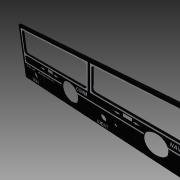
# Autodesk Inventor part: NavCom_panel
Saved by Autodesk Inventor 2014 (Build 180170000, 170)
## iProperties
Created: 2017-02-12
Part Number: NavCom_panel
Material: Všeobecné
Document SubType Name: Modeling
Designer: N
Density: 1 g/cm^3
Appearance: Výchozí
Author: N
Autodesk Inventor part; units mm, degrees
ref_plane "YZ Plane" through (0, 0, 0) normal (1, 0, 0) x (0, 1, 0)
ref_plane "XZ Plane" through (0, 0, 0) normal (0, 1, 0) x (-1, 0, 0)
ref_plane "XY Plane" through (0, 0, 0) normal (0, 0, 1) x (1, 0, 0)
sketch "Náčrt1" plane through (0, 0, 0) normal (0, 0, 1) x (1, 0, 0)
  circle A0 centre (29.21, 8.89) radius 2.54
  circle A1 centre (16.51, 8.89) radius 3.81
  circle A2 centre (65.405, 13.97) radius 10.795
  circle A3 centre (116.84, 8.89) radius 2.54
  circle A4 centre (104.14, 8.89) radius 3.81
  circle A5 centre (153.035, 13.97) radius 10.795
  line L0 (34.29, 25.7175) -> (44.45, 25.7175)
  line L1 (44.45, 25.7175) -> (44.45, 20.0025)
  line L2 (44.45, 20.0025) -> (34.29, 20.0025)
  line L3 (34.29, 20.0025) -> (34.29, 25.7175)
  line L4 (121.92, 25.7175) -> (132.08, 25.7175)
  line L5 (132.08, 25.7175) -> (132.08, 20.0025)
  line L6 (132.08, 20.0025) -> (121.92, 20.0025)
  line L7 (121.92, 20.0025) -> (121.92, 25.7175)
  line L8 (0, 55.88) -> (177.8, 55.88)
  line L9 (177.8, 55.88) -> (177.8, 0)
  line L10 (177.8, 0) -> (0, 0)
  line L11 (0, 0) -> (0, 55.88)
  line L12 (93.98, 52.07) -> (171.45, 52.07)
  arc A6 (173.99, 49.53) -> (171.45, 52.07) centre (171.45, 49.53) ccw
  line L13 (173.99, 49.53) -> (173.99, 30.48)
  arc A7 (171.45, 27.94) -> (173.99, 30.48) centre (171.45, 30.48) ccw
  line L14 (171.45, 27.94) -> (93.98, 27.94)
  arc A8 (91.44, 30.48) -> (93.98, 27.94) centre (93.98, 30.48) ccw
  line L15 (91.44, 30.48) -> (91.44, 49.53)
  arc A9 (93.98, 52.07) -> (91.44, 49.53) centre (93.98, 49.53) ccw
  line L16 (6.35, 52.07) -> (83.82, 52.07)
  arc A10 (86.36, 49.53) -> (83.82, 52.07) centre (83.82, 49.53) ccw
  line L17 (86.36, 49.53) -> (86.36, 30.48)
  arc A11 (83.82, 27.94) -> (86.36, 30.48) centre (83.82, 30.48) ccw
  line L18 (83.82, 27.94) -> (6.35, 27.94)
  arc A12 (3.81, 30.48) -> (6.35, 27.94) centre (6.35, 30.48) ccw
  line L19 (3.81, 30.48) -> (3.81, 49.53)
  arc A13 (6.35, 52.07) -> (3.81, 49.53) centre (6.35, 49.53) ccw
  constraints: 40 end point, 16 point on circle, 14 centre point
extrude "Vysunutí1" add sketch "Náčrt1" along normal blind 2.54
sketch "Náčrt2" plane through (0, 0, 2.54) normal (0, 0, 1) x (1, 0, 0)
  arc A0 (86.36, 49.53) -> (83.82, 52.07) centre (83.82, 49.53) ccw projected
  line L0 (86.36, 49.53) -> (86.36, 30.48) projected
  arc A1 (83.82, 27.94) -> (86.36, 30.48) centre (83.82, 30.48) ccw projected
  line L1 (83.82, 27.94) -> (6.35, 27.94) projected
  arc A2 (3.81, 30.48) -> (6.35, 27.94) centre (6.35, 30.48) ccw projected
  line L2 (3.81, 30.48) -> (3.81, 49.53) projected
  arc A3 (6.35, 52.07) -> (3.81, 49.53) centre (6.35, 49.53) ccw projected
  line L3 (6.35, 52.07) -> (83.82, 52.07) projected
  arc A4 (173.99, 49.53) -> (171.45, 52.07) centre (171.45, 49.53) ccw projected
  line L4 (173.99, 49.53) -> (173.99, 30.48) projected
  arc A5 (171.45, 27.94) -> (173.99, 30.48) centre (171.45, 30.48) ccw projected
  line L5 (171.45, 27.94) -> (93.98, 27.94) projected
  arc A6 (91.44, 30.48) -> (93.98, 27.94) centre (93.98, 30.48) ccw projected
  line L6 (91.44, 30.48) -> (91.44, 49.53) projected
  arc A7 (93.98, 52.07) -> (91.44, 49.53) centre (93.98, 49.53) ccw projected
  line L7 (93.98, 52.07) -> (171.45, 52.07) projected
  line L8 (0, 55.88) -> (177.8, 55.88)
  line L9 (177.8, 55.88) -> (177.8, 0)
  line L10 (177.8, 0) -> (0, 0)
  line L11 (0, 0) -> (0, 55.88)
  line L12 (74.93, 19.05) -> (143.51, 19.05)
  line L13 (162.56, 19.05) -> (171.45, 19.05)
  arc A8 (171.45, 19.05) -> (173.99, 21.59) centre (171.45, 21.59) ccw
  arc A9 (3.81, 21.59) -> (6.35, 19.05) centre (6.35, 21.59) ccw
  line L14 (87.63, 53.34) -> (2.54, 53.34)
  line L15 (6.35, 26.67) -> (87.63, 26.67)
  line L16 (2.54, 17.78) -> (2.54, 53.34)
  line L17 (3.81, 24.13) -> (3.81, 21.59)
  arc A10 (6.35, 26.67) -> (3.81, 24.13) centre (6.35, 24.13) ccw
  line L18 (90.17, 26.67) -> (171.45, 26.67)
  line L19 (175.26, 53.34) -> (90.17, 53.34)
  line L20 (90.17, 26.67) -> (90.17, 53.34)
  line L21 (87.63, 26.67) -> (87.63, 53.34)
  line L22 (175.26, 17.78) -> (175.26, 53.34)
  line L23 (173.99, 24.13) -> (173.99, 21.59)
  arc A11 (173.99, 24.13) -> (171.45, 26.67) centre (171.45, 24.13) ccw
  line L24 (175.26, 17.78) -> (163.1353, 17.78)
  line L25 (142.9347, 17.78) -> (75.5053, 17.78)
  line L26 (55.3047, 17.78) -> (2.54, 17.78)
  line L27 (6.35, 19.05) -> (55.88, 19.05)
  line L28 (93.98, 52.07) -> (171.45, 52.07)
  arc A12 (173.99, 49.53) -> (171.45, 52.07) centre (171.45, 49.53) ccw
  line L29 (173.99, 49.53) -> (173.99, 30.48)
  arc A13 (171.45, 27.94) -> (173.99, 30.48) centre (171.45, 30.48) ccw
  line L30 (171.45, 27.94) -> (93.98, 27.94)
  arc A14 (91.44, 30.48) -> (93.98, 27.94) centre (93.98, 30.48) ccw
  line L31 (91.44, 30.48) -> (91.44, 49.53)
  arc A15 (93.98, 52.07) -> (91.44, 49.53) centre (93.98, 49.53) ccw
  line L32 (6.35, 52.07) -> (83.82, 52.07)
  arc A16 (86.36, 49.53) -> (83.82, 52.07) centre (83.82, 49.53) ccw
  line L33 (86.36, 49.53) -> (86.36, 30.48)
  arc A17 (83.82, 27.94) -> (86.36, 30.48) centre (83.82, 30.48) ccw
  line L34 (83.82, 27.94) -> (6.35, 27.94)
  arc A18 (3.81, 30.48) -> (6.35, 27.94) centre (6.35, 30.48) ccw
  line L35 (3.81, 30.48) -> (3.81, 49.53)
  arc A19 (6.35, 52.07) -> (3.81, 49.53) centre (6.35, 49.53) ccw
  arc A20 (163.1353, 17.78) -> (162.56, 19.05) centre (153.035, 13.97) ccw
  arc A21 (143.51, 19.05) -> (142.9347, 17.78) centre (153.035, 13.97) ccw
  arc A22 (75.5053, 17.78) -> (74.93, 19.05) centre (65.405, 13.97) ccw
  arc A23 (55.88, 19.05) -> (55.3047, 17.78) centre (65.405, 13.97) ccw
  line L36 (29.02, 23.3287) -> (33.02, 23.3287)
  line L37 (31.52, 23.7975) -> (26.52, 22.86)
  line L38 (26.52, 22.86) -> (31.52, 21.9225)
  line L39 (29.02, 22.3913) -> (33.02, 22.3913)
  line L40 (31.52, 23.7975) -> (31.52, 21.9225)
  line L41 (33.02, 23.3287) -> (33.02, 22.3913)
  line L42 (49.72, 22.3913) -> (45.72, 22.3913)
  line L43 (47.22, 21.9225) -> (52.22, 22.86)
  line L44 (52.22, 22.86) -> (47.22, 23.7975)
  line L45 (49.72, 23.3287) -> (45.72, 23.3287)
  line L46 (47.22, 21.9225) -> (47.22, 23.7975)
  line L47 (45.72, 22.3913) -> (45.72, 23.3287)
  line L48 (137.337, 22.4606) -> (133.337, 22.4606)
  line L49 (134.837, 21.9919) -> (139.837, 22.9294)
  line L50 (139.837, 22.9294) -> (134.837, 23.8669)
  line L51 (137.337, 23.3981) -> (133.337, 23.3981)
  line L52 (134.837, 21.9919) -> (134.837, 23.8669)
  line L53 (133.337, 22.4606) -> (133.337, 23.3981)
  line L54 (116.65, 23.3287) -> (120.65, 23.3287)
  line L55 (119.15, 23.7975) -> (114.15, 22.86)
  line L56 (114.15, 22.86) -> (119.15, 21.9225)
  line L57 (116.65, 22.3913) -> (120.65, 22.3913)
  line L58 (119.15, 23.7975) -> (119.15, 21.9225)
  line L59 (120.65, 23.3287) -> (120.65, 22.3913)
  line L60 (163.9202, 21.265) -> (163.9202, 24.765)
  line L61 (163.9202, 24.765) -> (164.4849, 24.765)
  line L62 (164.4849, 24.765) -> (165.6579, 22.4271)
  line L63 (165.6579, 22.4271) -> (165.6579, 24.765)
  line L64 (165.6579, 24.765) -> (166.198, 24.765)
  line L65 (166.198, 24.765) -> (166.198, 21.265)
  line L66 (166.198, 21.265) -> (165.6142, 21.265)
  line L67 (165.6142, 21.265) -> (164.4603, 23.5483)
  line L68 (164.4603, 23.5483) -> (164.4603, 21.265)
  line L69 (164.4603, 21.265) -> (163.9202, 21.265)
  line L70 (169.3952, 21.265) -> (168.7678, 21.265)
  line L71 (168.7678, 21.265) -> (168.5168, 22.0588)
  line L72 (168.5168, 22.0588) -> (167.3711, 22.0588)
  line L73 (167.3711, 22.0588) -> (167.1337, 21.265)
  line L74 (167.1337, 21.265) -> (166.5172, 21.265)
  line L75 (166.5172, 21.265) -> (167.6302, 24.765)
  line L76 (167.6302, 24.765) -> (168.2495, 24.765)
  line L77 (168.2495, 24.765) -> (169.3952, 21.265)
  line L78 (168.3313, 22.6508) -> (167.9357, 23.9493)
  line L79 (167.9357, 23.9493) -> (167.5456, 22.6508)
  line L80 (167.5456, 22.6508) -> (168.3313, 22.6508)
  line L81 (170.4346, 21.265) -> (169.4116, 24.765)
  line L82 (169.4116, 24.765) -> (170.039, 24.765)
  line L83 (170.039, 24.765) -> (170.7674, 22.1734)
  line L84 (170.7674, 22.1734) -> (171.4685, 24.765)
  line L85 (171.4685, 24.765) -> (172.085, 24.765)
  line L86 (172.085, 24.765) -> (171.0566, 21.265)
  line L87 (171.0566, 21.265) -> (170.4346, 21.265)
  line L88 (98.7379, 1.27) -> (98.7379, 4.77)
  line L89 (98.7379, 4.77) -> (99.3162, 4.77)
  line L90 (99.3162, 4.77) -> (99.3162, 1.27)
  line L91 (99.3162, 1.27) -> (98.7379, 1.27)
  line L92 (99.8673, 4.77) -> (100.923, 4.77)
  spline S0 degree 2 poles (100.923, 4.77) (101.324, 4.77) (101.7305, 4.5899) (102.0742, 4.1671) (102.2706, 3.4878) (102.2706, 2.9832) knots 0 0 0 1 2 3 4 4 4
  spline S1 degree 2 poles (102.2706, 2.9832) (102.2706, 2.5303) (102.066, 1.8592) (101.7496, 1.4691) (101.3049, 1.27) (100.9557, 1.27) knots 0 0 0 1 2 3 4 4 4
  line L93 (100.9557, 1.27) -> (99.8673, 1.27)
  line L94 (99.8673, 1.27) -> (99.8673, 4.77)
  line L95 (100.4456, 4.178) -> (100.4456, 1.862)
  line L96 (100.4456, 1.862) -> (100.8793, 1.862)
  spline S2 degree 2 poles (100.8793, 1.862) (101.1576, 1.862) (101.4086, 1.9656) (101.5695, 2.1784) (101.6732, 2.6367) (101.6732, 3.0104) knots 0 0 0 1 2 3 4 4 4
  spline S3 degree 2 poles (101.6732, 3.0104) (101.6732, 3.4005) (101.5668, 3.8479) (101.3404, 4.1071) (101.1767, 4.148) knots 0 0 0 1 2 3 3 3
  spline S4 degree 2 poles (101.1767, 4.148) (101.0567, 4.178) (100.7075, 4.178) knots 0 0 0 1 1 1
  line L97 (100.7075, 4.178) -> (100.4456, 4.178)
  line L98 (102.7671, 1.27) -> (102.7671, 4.77)
  line L99 (102.7671, 4.77) -> (104.8976, 4.77)
  line L100 (104.8976, 4.77) -> (104.8976, 4.178)
  line L101 (104.8976, 4.178) -> (103.3454, 4.178)
  line L102 (103.3454, 4.178) -> (103.3454, 3.4005)
  line L103 (103.3454, 3.4005) -> (104.7885, 3.4005)
  line L104 (104.7885, 3.4005) -> (104.7885, 2.8113)
  line L105 (104.7885, 2.8113) -> (103.3454, 2.8113)
  line L106 (103.3454, 2.8113) -> (103.3454, 1.862)
  line L107 (103.3454, 1.862) -> (104.9495, 1.862)
  line L108 (104.9495, 1.862) -> (104.9495, 1.27)
  line L109 (104.9495, 1.27) -> (102.7671, 1.27)
  line L110 (105.4432, 1.27) -> (105.4432, 4.77)
  line L111 (105.4432, 4.77) -> (106.0079, 4.77)
  line L112 (106.0079, 4.77) -> (107.181, 2.4321)
  line L113 (107.181, 2.4321) -> (107.181, 4.77)
  line L114 (107.181, 4.77) -> (107.7211, 4.77)
  line L115 (107.7211, 4.77) -> (107.7211, 1.27)
  line L116 (107.7211, 1.27) -> (107.1373, 1.27)
  line L117 (107.1373, 1.27) -> (105.9834, 3.5533)
  line L118 (105.9834, 3.5533) -> (105.9834, 1.27)
  line L119 (105.9834, 1.27) -> (105.4432, 1.27)
  line L120 (108.9787, 1.27) -> (108.9787, 4.178)
  line L121 (108.9787, 4.178) -> (108.1276, 4.178)
  line L122 (108.1276, 4.178) -> (108.1276, 4.77)
  line L123 (108.1276, 4.77) -> (110.4082, 4.77)
  line L124 (110.4082, 4.77) -> (110.4082, 4.178)
  line L125 (110.4082, 4.178) -> (109.557, 4.178)
  line L126 (109.557, 4.178) -> (109.557, 1.27)
  line L127 (109.557, 1.27) -> (108.9787, 1.27)
  line L128 (12.2821, 1.33) -> (12.2821, 4.238)
  line L129 (12.2821, 4.238) -> (11.431, 4.238)
  line L130 (11.431, 4.238) -> (11.431, 4.83)
  line L131 (11.431, 4.83) -> (13.7116, 4.83)
  line L132 (13.7116, 4.83) -> (13.7116, 4.238)
  line L133 (13.7116, 4.238) -> (12.8605, 4.238)
  line L134 (12.8605, 4.238) -> (12.8605, 1.33)
  line L135 (12.8605, 1.33) -> (12.2821, 1.33)
  line L136 (14.0881, 1.33) -> (14.0881, 4.83)
  line L137 (14.0881, 4.83) -> (16.2186, 4.83)
  line L138 (16.2186, 4.83) -> (16.2186, 4.238)
  line L139 (16.2186, 4.238) -> (14.6664, 4.238)
  line L140 (14.6664, 4.238) -> (14.6664, 3.4606)
  line L141 (14.6664, 3.4606) -> (16.1095, 3.4606)
  line L142 (16.1095, 3.4606) -> (16.1095, 2.8713)
  line L143 (16.1095, 2.8713) -> (14.6664, 2.8713)
  line L144 (14.6664, 2.8713) -> (14.6664, 1.922)
  line L145 (14.6664, 1.922) -> (16.2704, 1.922)
  line L146 (16.2704, 1.922) -> (16.2704, 1.33)
  line L147 (16.2704, 1.33) -> (14.0881, 1.33)
  line L148 (16.6142, 2.4703) -> (17.1789, 2.5385)
  spline S5 degree 2 poles (17.1789, 2.5385) (17.2743, 1.8674) (17.8036, 1.8674) knots 0 0 0 1 1 1
  spline S6 degree 2 poles (17.8036, 1.8674) (18.0655, 1.8674) (18.3655, 2.143) (18.3655, 2.3448) knots 0 0 0 1 2 2 2
  spline S7 degree 2 poles (18.3655, 2.3448) (18.3655, 2.4649) (18.2619, 2.6313) (18.0464, 2.7377) (17.6344, 2.8659) knots 0 0 0 1 2 3 3 3
  spline S8 degree 2 poles (17.6344, 2.8659) (17.2634, 2.9777) (16.9197, 3.2396) (16.7178, 3.6652) (16.7178, 3.9107) knots 0 0 0 1 2 3 3 3
  spline S9 degree 2 poles (16.7178, 3.9107) (16.7178, 4.1971) (16.977, 4.6554) (17.438, 4.89) (17.7736, 4.89) knots 0 0 0 1 2 3 3 3
  spline S10 degree 2 poles (17.7736, 4.89) (18.281, 4.89) (18.8484, 4.339) (18.8648, 3.8288) knots 0 0 0 1 2 2 2
  line L149 (18.8648, 3.8288) -> (18.2837, 3.7988)
  spline S11 degree 2 poles (18.2837, 3.7988) (18.2455, 4.0825) (17.9918, 4.3062) (17.7599, 4.3062) knots 0 0 0 1 2 2 2
  spline S12 degree 2 poles (17.7599, 4.3062) (17.5253, 4.3062) (17.2716, 4.1098) (17.2716, 3.9652) knots 0 0 0 1 2 2 2
  spline S13 degree 2 poles (17.2716, 3.9652) (17.2716, 3.8234) (17.3862, 3.7252) knots 0 0 0 1 1 1
  spline S14 degree 2 poles (17.3862, 3.7252) (17.5008, 3.627) (17.9127, 3.5097) knots 0 0 0 1 1 1
  spline S15 degree 2 poles (17.9127, 3.5097) (18.3492, 3.3842) (18.7393, 3.1032) (18.9439, 2.6613) (18.9439, 2.3476) knots 0 0 0 1 2 3 3 3
  spline S16 degree 2 poles (18.9439, 2.3476) (18.9439, 1.892) (18.3846, 1.27) (17.7872, 1.27) knots 0 0 0 1 2 2 2
  spline S17 degree 2 poles (17.7872, 1.27) (16.7342, 1.27) (16.6142, 2.4703) knots 0 0 0 1 1 1
  line L150 (20.0787, 1.33) -> (20.0787, 4.238)
  line L151 (20.0787, 4.238) -> (19.2276, 4.238)
  line L152 (19.2276, 4.238) -> (19.2276, 4.83)
  line L153 (19.2276, 4.83) -> (21.5082, 4.83)
  line L154 (21.5082, 4.83) -> (21.5082, 4.238)
  line L155 (21.5082, 4.238) -> (20.657, 4.238)
  line L156 (20.657, 4.238) -> (20.657, 1.33)
  line L157 (20.657, 1.33) -> (20.0787, 1.33)
  line L158 (5.6925, 14.6398) -> (5.3342, 14.6398)
  line L159 (5.3342, 14.6398) -> (5.0384, 16.6398)
  line L160 (5.0384, 16.6398) -> (5.3733, 16.6398)
  line L161 (5.3733, 16.6398) -> (5.5846, 15.1265)
  line L162 (5.5846, 15.1265) -> (6.2638, 16.6398)
  line L163 (6.2638, 16.6398) -> (6.5955, 16.6398)
  line L164 (6.5955, 16.6398) -> (5.6925, 14.6398)
  line L165 (7.5548, 15.2423) -> (6.7489, 15.2423)
  line L166 (6.7489, 15.2423) -> (6.7489, 15.2063)
  spline S18 degree 2 poles (6.7489, 15.2063) (6.7489, 15.0592) (6.885, 14.8855) (6.9805, 14.8855) knots 0 0 0 1 2 2 2
  spline S19 degree 2 poles (6.9805, 14.8855) (7.1386, 14.8855) (7.2293, 15.0874) knots 0 0 0 1 1 1
  line L167 (7.2293, 15.0874) -> (7.5173, 15.0295)
  spline S20 degree 2 poles (7.5173, 15.0295) (7.4328, 14.8182) (7.1526, 14.607) (6.9774, 14.607) knots 0 0 0 1 2 2 2
  spline S21 degree 2 poles (6.9774, 14.607) (6.7458, 14.607) (6.439, 14.9685) (6.439, 15.2783) knots 0 0 0 1 2 2 2
  spline S22 degree 2 poles (6.439, 15.2783) (6.439, 15.6132) (6.788, 16.1218) (7.1026, 16.1218) knots 0 0 0 1 2 2 2
  spline S23 degree 2 poles (7.1026, 16.1218) (7.3138, 16.1218) (7.5767, 15.801) (7.5767, 15.4974) knots 0 0 0 1 2 2 2
  spline S24 degree 2 poles (7.5767, 15.4974) (7.5767, 15.355) (7.5548, 15.2423) knots 0 0 0 1 1 1
  line L168 (7.2825, 15.4818) -> (7.2841, 15.5193)
  spline S25 degree 2 poles (7.2841, 15.5193) (7.2841, 15.6852) (7.1636, 15.8433) (7.0666, 15.8433) knots 0 0 0 1 2 2 2
  spline S26 degree 2 poles (7.0666, 15.8433) (6.968, 15.8433) (6.8084, 15.6602) (6.7817, 15.4818) knots 0 0 0 1 2 2 2
  line L169 (6.7817, 15.4818) -> (7.2825, 15.4818)
  line L170 (7.8944, 16.089) -> (8.1965, 16.089)
  line L171 (8.1965, 16.089) -> (8.1495, 15.8073)
  spline S27 degree 2 poles (8.1495, 15.8073) (8.317, 16.1218) (8.5157, 16.1218) knots 0 0 0 1 1 1
  spline S28 degree 2 poles (8.5157, 16.1218) (8.5846, 16.1218) (8.6659, 16.0812) knots 0 0 0 1 1 1
  line L172 (8.6659, 16.0812) -> (8.5423, 15.7603)
  spline S29 degree 2 poles (8.5423, 15.7603) (8.4985, 15.7791) (8.45, 15.7791) knots 0 0 0 1 1 1
  spline S30 degree 2 poles (8.45, 15.7791) (8.3749, 15.7791) (8.3076, 15.729) knots 0 0 0 1 1 1
  spline S31 degree 2 poles (8.3076, 15.729) (8.2074, 15.6508) (8.0994, 15.4004) (8.0478, 15.0937) knots 0 0 0 1 2 2 2
  line L173 (8.0478, 15.0937) -> (7.968, 14.6398)
  line L174 (7.968, 14.6398) -> (7.6456, 14.6398)
  line L175 (7.6456, 14.6398) -> (7.8944, 16.089)
  line L176 (8.536, 14.6398) -> (8.8788, 16.6398)
  line L177 (8.8788, 16.6398) -> (9.2011, 16.6398)
  line L178 (9.2011, 16.6398) -> (9.0869, 15.9716)
  spline S32 degree 2 poles (9.0869, 15.9716) (9.1808, 16.0577) (9.3295, 16.1218) (9.4155, 16.1218) knots 0 0 0 1 2 2 2
  spline S33 degree 2 poles (9.4155, 16.1218) (9.6018, 16.1218) (9.8303, 15.8182) (9.8303, 15.5209) knots 0 0 0 1 2 2 2
  spline S34 degree 2 poles (9.8303, 15.5209) (9.8303, 15.2502) (9.6519, 14.8151) (9.3827, 14.607) (9.2434, 14.607) knots 0 0 0 1 2 3 3 3
  spline S35 degree 2 poles (9.2434, 14.607) (8.9883, 14.607) (8.8694, 14.8761) knots 0 0 0 1 1 1
  line L179 (8.8694, 14.8761) -> (8.8287, 14.6398)
  line L180 (8.8287, 14.6398) -> (8.536, 14.6398)
  spline S36 degree 2 poles (8.9695, 15.2298) (8.9695, 15.0796) (9.1057, 14.8996) (9.1949, 14.8996) knots 0 0 0 1 2 2 2
  spline S37 degree 2 poles (9.1949, 14.8996) (9.2669, 14.8996) (9.4093, 15.0217) (9.5173, 15.3378) (9.5173, 15.5115) knots 0 0 0 1 2 3 3 3
  spline S38 degree 2 poles (9.5173, 15.5115) (9.5173, 15.6711) (9.3858, 15.8433) (9.295, 15.8433) knots 0 0 0 1 2 2 2
  spline S39 degree 2 poles (9.295, 15.8433) (9.1558, 15.8433) (8.9695, 15.4818) (8.9695, 15.2298) knots 0 0 0 1 2 2 2
  line L181 (10.414, 15.6774) -> (10.101, 15.7103)
  spline S40 degree 2 poles (10.101, 15.7103) (10.1573, 15.9106) (10.4343, 16.1218) (10.6472, 16.1218) knots 0 0 0 1 2 2 2
  spline S41 degree 2 poles (10.6472, 16.1218) (10.8647, 16.1218) (11.0979, 15.9074) (11.0979, 15.729) knots 0 0 0 1 2 2 2
  spline S42 degree 2 poles (11.0979, 15.729) (11.0979, 15.6664) (11.0759, 15.5256) (11.0055, 15.211) knots 0 0 0 1 2 2 2
  spline S43 degree 2 poles (11.0055, 15.211) (10.9461, 14.9513) (10.9461, 14.848) knots 0 0 0 1 1 1
  spline S44 degree 2 poles (10.9461, 14.848) (10.9461, 14.7525) (10.9789, 14.6398) knots 0 0 0 1 1 1
  line L182 (10.9789, 14.6398) -> (10.6581, 14.6398)
  spline S45 degree 2 poles (10.6581, 14.6398) (10.6393, 14.7197) (10.6346, 14.8042) knots 0 0 0 1 1 1
  spline S46 degree 2 poles (10.6346, 14.8042) (10.5658, 14.7087) (10.3889, 14.607) (10.3013, 14.607) knots 0 0 0 1 2 2 2
  spline S47 degree 2 poles (10.3013, 14.607) (10.162, 14.607) (9.9727, 14.8355) (9.9727, 15.0279) knots 0 0 0 1 2 2 2
  spline S48 degree 2 poles (9.9727, 15.0279) (9.9727, 15.247) (10.0838, 15.366) knots 0 0 0 1 1 1
  spline S49 degree 2 poles (10.0838, 15.366) (10.1949, 15.4849) (10.4547, 15.5084) knots 0 0 0 1 1 1
  spline S50 degree 2 poles (10.4547, 15.5084) (10.6847, 15.5319) (10.7614, 15.5647) knots 0 0 0 1 1 1
  spline S51 degree 2 poles (10.7614, 15.5647) (10.788, 15.6477) (10.788, 15.6962) knots 0 0 0 1 1 1
  spline S52 degree 2 poles (10.788, 15.6962) (10.788, 15.7619) (10.6972, 15.8433) (10.6206, 15.8433) knots 0 0 0 1 2 2 2
  spline S53 degree 2 poles (10.6206, 15.8433) (10.4515, 15.8433) (10.414, 15.6774) knots 0 0 0 1 1 1
  spline S54 degree 2 poles (10.7098, 15.3143) (10.68, 15.3049) (10.6331, 15.2971) knots 0 0 0 1 1 1
  spline S55 degree 2 poles (10.6331, 15.2971) (10.414, 15.2643) (10.2747, 15.1531) (10.2747, 15.0608) knots 0 0 0 1 2 2 2
  spline S56 degree 2 poles (10.2747, 15.0608) (10.2747, 14.9888) (10.3545, 14.8996) (10.4155, 14.8996) knots 0 0 0 1 2 2 2
  spline S57 degree 2 poles (10.4155, 14.8996) (10.4781, 14.8996) (10.5955, 14.9747) (10.6644, 15.1093) (10.6972, 15.2627) knots 0 0 0 1 2 3 3 3
  line L183 (10.6972, 15.2627) -> (10.7098, 15.3143)
  line L184 (13.0634, 15.3597) -> (13.403, 15.2987)
  spline S58 degree 2 poles (13.403, 15.2987) (13.3013, 14.9513) (12.9007, 14.6054) (12.6378, 14.6054) knots 0 0 0 1 2 2 2
  spline S59 degree 2 poles (12.6378, 14.6054) (12.3436, 14.6054) (11.9977, 15.0358) (11.9977, 15.4677) knots 0 0 0 1 2 2 2
  spline S60 degree 2 poles (11.9977, 15.4677) (11.9977, 15.837) (12.2481, 16.4004) (12.6378, 16.6743) (12.8647, 16.6743) knots 0 0 0 1 2 3 3 3
  spline S61 degree 2 poles (12.8647, 16.6743) (13.1198, 16.6743) (13.4594, 16.3378) (13.4891, 16.0248) knots 0 0 0 1 2 2 2
  line L185 (13.4891, 16.0248) -> (13.1651, 15.9873)
  spline S62 degree 2 poles (13.1651, 15.9873) (13.137, 16.1688) (12.982, 16.319) (12.8584, 16.319) knots 0 0 0 1 2 2 2
  spline S63 degree 2 poles (12.8584, 16.319) (12.7317, 16.319) (12.4969, 16.1359) (12.3326, 15.7071) (12.3326, 15.4489) knots 0 0 0 1 2 3 3 3
  spline S64 degree 2 poles (12.3326, 15.4489) (12.3326, 15.2079) (12.5235, 14.9497) (12.6597, 14.9497) knots 0 0 0 1 2 2 2
  spline S65 degree 2 poles (12.6597, 14.9497) (12.788, 14.9497) (13.0087, 15.1531) (13.0634, 15.3597) knots 0 0 0 1 2 2 2
  spline S66 degree 2 poles (13.5736, 15.2423) (13.5736, 15.5976) (13.7348, 15.848) knots 0 0 0 1 1 1
  spline S67 degree 2 poles (13.7348, 15.848) (13.9132, 16.1218) (14.2512, 16.1218) knots 0 0 0 1 1 1
  spline S68 degree 2 poles (14.2512, 16.1218) (14.5047, 16.1218) (14.8068, 15.7776) (14.8068, 15.4708) knots 0 0 0 1 2 2 2
  spline S69 degree 2 poles (14.8068, 15.4708) (14.8068, 15.1109) (14.4312, 14.607) (14.1292, 14.607) knots 0 0 0 1 2 2 2
  spline S70 degree 2 poles (14.1292, 14.607) (13.8819, 14.607) (13.5736, 14.9481) (13.5736, 15.2423) knots 0 0 0 1 2 2 2
  spline S71 degree 2 poles (14.4891, 15.5225) (14.4891, 15.6649) (14.3545, 15.8292) (14.2497, 15.8292) knots 0 0 0 1 2 2 2
  spline S72 degree 2 poles (14.2497, 15.8292) (14.162, 15.8292) (14.0087, 15.7087) (13.8944, 15.4114) (13.8944, 15.2517) knots 0 0 0 1 2 3 3 3
  spline S73 degree 2 poles (13.8944, 15.2517) (13.8944, 15.089) (14.0353, 14.909) (14.1385, 14.909) knots 0 0 0 1 2 2 2
  spline S74 degree 2 poles (14.1385, 14.909) (14.27, 14.909) (14.3623, 15.0483) knots 0 0 0 1 1 1
  spline S75 degree 2 poles (14.3623, 15.0483) (14.4891, 15.2392) (14.4891, 15.5225) knots 0 0 0 1 1 1
  line L186 (15.1464, 16.089) -> (15.4484, 16.089)
  line L187 (15.4484, 16.089) -> (15.4014, 15.8073)
  spline S76 degree 2 poles (15.4014, 15.8073) (15.5689, 16.1218) (15.7676, 16.1218) knots 0 0 0 1 1 1
  spline S77 degree 2 poles (15.7676, 16.1218) (15.8365, 16.1218) (15.9179, 16.0812) knots 0 0 0 1 1 1
  line L188 (15.9179, 16.0812) -> (15.7942, 15.7603)
  spline S78 degree 2 poles (15.7942, 15.7603) (15.7504, 15.7791) (15.7019, 15.7791) knots 0 0 0 1 1 1
  spline S79 degree 2 poles (15.7019, 15.7791) (15.6268, 15.7791) (15.5595, 15.729) knots 0 0 0 1 1 1
  spline S80 degree 2 poles (15.5595, 15.729) (15.4594, 15.6508) (15.3514, 15.4004) (15.2997, 15.0937) knots 0 0 0 1 2 2 2
  line L189 (15.2997, 15.0937) -> (15.2199, 14.6398)
  line L190 (15.2199, 14.6398) -> (14.8975, 14.6398)
  line L191 (14.8975, 14.6398) -> (15.1464, 16.089)
  line L192 (16.0493, 16.089) -> (16.3561, 16.089)
  line L193 (16.3561, 16.089) -> (16.331, 15.9403)
  spline S81 degree 2 poles (16.331, 15.9403) (16.4312, 16.042) (16.5955, 16.1218) (16.6863, 16.1218) knots 0 0 0 1 2 2 2
  spline S82 degree 2 poles (16.6863, 16.1218) (16.8662, 16.1218) (17.09, 15.8104) (17.09, 15.4974) knots 0 0 0 1 2 2 2
  spline S83 degree 2 poles (17.09, 15.4974) (17.09, 15.0999) (16.8913, 14.8292) knots 0 0 0 1 1 1
  spline S84 degree 2 poles (16.8913, 14.8292) (16.7285, 14.607) (16.5079, 14.607) knots 0 0 0 1 1 1
  spline S85 degree 2 poles (16.5079, 14.607) (16.2778, 14.607) (16.1589, 14.837) knots 0 0 0 1 1 1
  line L194 (16.1589, 14.837) -> (16.0274, 14.0874)
  line L195 (16.0274, 14.0874) -> (15.7066, 14.0874)
  line L196 (15.7066, 14.0874) -> (16.0493, 16.089)
  spline S86 degree 2 poles (16.245, 15.2564) (16.245, 15.0858) (16.3764, 14.8996) (16.464, 14.8996) knots 0 0 0 1 2 2 2
  spline S87 degree 2 poles (16.464, 14.8996) (16.5329, 14.8996) (16.6675, 15.0186) (16.777, 15.3394) (16.777, 15.5084) knots 0 0 0 1 2 3 3 3
  spline S88 degree 2 poles (16.777, 15.5084) (16.777, 15.6711) (16.6518, 15.8433) (16.5595, 15.8433) knots 0 0 0 1 2 2 2
  spline S89 degree 2 poles (16.5595, 15.8433) (16.4875, 15.8433) (16.3514, 15.7259) (16.245, 15.4192) (16.245, 15.2564) knots 0 0 0 1 2 3 3 3
  line L197 (17.2888, 15.017) -> (17.6049, 15.017)
  line L198 (17.6049, 15.017) -> (17.5392, 14.6398)
  line L199 (17.5392, 14.6398) -> (17.223, 14.6398)
  line L200 (17.223, 14.6398) -> (17.2888, 15.017)
  line L201 (24.2559, 14.6398) -> (23.9413, 14.6398)
  line L202 (23.9413, 14.6398) -> (23.5, 15.9841)
  line L203 (23.5, 15.9841) -> (23.27, 14.6398)
  line L204 (23.27, 14.6398) -> (22.9554, 14.6398)
  line L205 (22.9554, 14.6398) -> (23.2981, 16.6398)
  line L206 (23.2981, 16.6398) -> (23.6127, 16.6398)
  line L207 (23.6127, 16.6398) -> (24.054, 15.3018)
  line L208 (24.054, 15.3018) -> (24.2841, 16.6398)
  line L209 (24.2841, 16.6398) -> (24.5986, 16.6398)
  line L210 (24.5986, 16.6398) -> (24.2559, 14.6398)
  line L211 (25.0509, 15.6774) -> (24.7379, 15.7103)
  spline S90 degree 2 poles (24.7379, 15.7103) (24.7942, 15.9106) (25.0712, 16.1218) (25.2841, 16.1218) knots 0 0 0 1 2 2 2
  spline S91 degree 2 poles (25.2841, 16.1218) (25.5016, 16.1218) (25.7348, 15.9074) (25.7348, 15.729) knots 0 0 0 1 2 2 2
  spline S92 degree 2 poles (25.7348, 15.729) (25.7348, 15.6664) (25.7129, 15.5256) (25.6424, 15.211) knots 0 0 0 1 2 2 2
  spline S93 degree 2 poles (25.6424, 15.211) (25.583, 14.9513) (25.583, 14.848) knots 0 0 0 1 1 1
  spline S94 degree 2 poles (25.583, 14.848) (25.583, 14.7525) (25.6158, 14.6398) knots 0 0 0 1 1 1
  line L212 (25.6158, 14.6398) -> (25.295, 14.6398)
  spline S95 degree 2 poles (25.295, 14.6398) (25.2762, 14.7197) (25.2715, 14.8042) knots 0 0 0 1 1 1
  spline S96 degree 2 poles (25.2715, 14.8042) (25.2027, 14.7087) (25.0258, 14.607) (24.9382, 14.607) knots 0 0 0 1 2 2 2
  spline S97 degree 2 poles (24.9382, 14.607) (24.7989, 14.607) (24.6096, 14.8355) (24.6096, 15.0279) knots 0 0 0 1 2 2 2
  spline S98 degree 2 poles (24.6096, 15.0279) (24.6096, 15.247) (24.7207, 15.366) knots 0 0 0 1 1 1
  spline S99 degree 2 poles (24.7207, 15.366) (24.8318, 15.4849) (25.0916, 15.5084) knots 0 0 0 1 1 1
  spline S100 degree 2 poles (25.0916, 15.5084) (25.3216, 15.5319) (25.3983, 15.5647) knots 0 0 0 1 1 1
  spline S101 degree 2 poles (25.3983, 15.5647) (25.4249, 15.6477) (25.4249, 15.6962) knots 0 0 0 1 1 1
  spline S102 degree 2 poles (25.4249, 15.6962) (25.4249, 15.7619) (25.3341, 15.8433) (25.2575, 15.8433) knots 0 0 0 1 2 2 2
  spline S103 degree 2 poles (25.2575, 15.8433) (25.0884, 15.8433) (25.0509, 15.6774) knots 0 0 0 1 1 1
  spline S104 degree 2 poles (25.3467, 15.3143) (25.3169, 15.3049) (25.27, 15.2971) knots 0 0 0 1 1 1
  spline S105 degree 2 poles (25.27, 15.2971) (25.0509, 15.2643) (24.9116, 15.1531) (24.9116, 15.0608) knots 0 0 0 1 2 2 2
  spline S106 degree 2 poles (24.9116, 15.0608) (24.9116, 14.9888) (24.9914, 14.8996) (25.0524, 14.8996) knots 0 0 0 1 2 2 2
  spline S107 degree 2 poles (25.0524, 14.8996) (25.115, 14.8996) (25.2324, 14.9747) (25.3013, 15.1093) (25.3341, 15.2627) knots 0 0 0 1 2 3 3 3
  line L213 (25.3341, 15.2627) -> (25.3467, 15.3143)
  line L214 (26.4687, 14.6398) -> (26.1917, 14.6398)
  line L215 (26.1917, 14.6398) -> (25.9523, 16.089)
  line L216 (25.9523, 16.089) -> (26.2668, 16.089)
  line L217 (26.2668, 16.089) -> (26.3513, 15.4567)
  spline S108 degree 2 poles (26.3513, 15.4567) (26.3842, 15.211) (26.3936, 15.1156) knots 0 0 0 1 1 1
  line L218 (26.3936, 15.1156) -> (26.464, 15.2768)
  line L219 (26.464, 15.2768) -> (26.5548, 15.4771)
  line L220 (26.5548, 15.4771) -> (26.849, 16.089)
  line L221 (26.849, 16.089) -> (27.1964, 16.089)
  line L222 (27.1964, 16.089) -> (26.4687, 14.6398)
  line L223 (26.9539, 14.607) -> (27.7661, 16.6743)
  line L224 (27.7661, 16.6743) -> (27.9914, 16.6743)
  line L225 (27.9914, 16.6743) -> (27.1792, 14.607)
  line L226 (27.1792, 14.607) -> (26.9539, 14.607)
  line L227 (28.9742, 15.3597) -> (29.3138, 15.2987)
  spline S109 degree 2 poles (29.3138, 15.2987) (29.2121, 14.9513) (28.8114, 14.6054) (28.5485, 14.6054) knots 0 0 0 1 2 2 2
  spline S110 degree 2 poles (28.5485, 14.6054) (28.2543, 14.6054) (27.9085, 15.0358) (27.9085, 15.4677) knots 0 0 0 1 2 2 2
  spline S111 degree 2 poles (27.9085, 15.4677) (27.9085, 15.837) (28.1589, 16.4004) (28.5485, 16.6743) (28.7754, 16.6743) knots 0 0 0 1 2 3 3 3
  spline S112 degree 2 poles (28.7754, 16.6743) (29.0305, 16.6743) (29.3701, 16.3378) (29.3999, 16.0248) knots 0 0 0 1 2 2 2
  line L228 (29.3999, 16.0248) -> (29.0759, 15.9873)
  spline S113 degree 2 poles (29.0759, 15.9873) (29.0477, 16.1688) (28.8928, 16.319) (28.7692, 16.319) knots 0 0 0 1 2 2 2
  spline S114 degree 2 poles (28.7692, 16.319) (28.6424, 16.319) (28.4077, 16.1359) (28.2434, 15.7071) (28.2434, 15.4489) knots 0 0 0 1 2 3 3 3
  spline S115 degree 2 poles (28.2434, 15.4489) (28.2434, 15.2079) (28.4343, 14.9497) (28.5704, 14.9497) knots 0 0 0 1 2 2 2
  spline S116 degree 2 poles (28.5704, 14.9497) (28.6988, 14.9497) (28.9194, 15.1531) (28.9742, 15.3597) knots 0 0 0 1 2 2 2
  spline S117 degree 2 poles (29.4844, 15.2423) (29.4844, 15.5976) (29.6456, 15.848) knots 0 0 0 1 1 1
  spline S118 degree 2 poles (29.6456, 15.848) (29.824, 16.1218) (30.162, 16.1218) knots 0 0 0 1 1 1
  spline S119 degree 2 poles (30.162, 16.1218) (30.4155, 16.1218) (30.7175, 15.7776) (30.7175, 15.4708) knots 0 0 0 1 2 2 2
  spline S120 degree 2 poles (30.7175, 15.4708) (30.7175, 15.1109) (30.342, 14.607) (30.0399, 14.607) knots 0 0 0 1 2 2 2
  spline S121 degree 2 poles (30.0399, 14.607) (29.7927, 14.607) (29.4844, 14.9481) (29.4844, 15.2423) knots 0 0 0 1 2 2 2
  spline S122 degree 2 poles (30.3999, 15.5225) (30.3999, 15.6649) (30.2653, 15.8292) (30.1604, 15.8292) knots 0 0 0 1 2 2 2
  spline S123 degree 2 poles (30.1604, 15.8292) (30.0728, 15.8292) (29.9194, 15.7087) (29.8052, 15.4114) (29.8052, 15.2517) knots 0 0 0 1 2 3 3 3
  spline S124 degree 2 poles (29.8052, 15.2517) (29.8052, 15.089) (29.946, 14.909) (30.0493, 14.909) knots 0 0 0 1 2 2 2
  spline S125 degree 2 poles (30.0493, 14.909) (30.1808, 14.909) (30.2731, 15.0483) knots 0 0 0 1 1 1
  spline S126 degree 2 poles (30.2731, 15.0483) (30.3999, 15.2392) (30.3999, 15.5225) knots 0 0 0 1 1 1
  line L229 (31.0571, 16.089) -> (31.3623, 16.089)
  line L230 (31.3623, 16.089) -> (31.331, 15.9137)
  spline S127 degree 2 poles (31.331, 15.9137) (31.511, 16.1218) (31.7081, 16.1218) knots 0 0 0 1 1 1
  spline S128 degree 2 poles (31.7081, 16.1218) (31.9711, 16.1218) (32.0133, 15.8668) knots 0 0 0 1 1 1
  spline S129 degree 2 poles (32.0133, 15.8668) (32.0775, 15.9779) (32.3122, 16.1218) (32.4311, 16.1218) knots 0 0 0 1 2 2 2
  spline S130 degree 2 poles (32.4311, 16.1218) (32.572, 16.1218) (32.7379, 15.9419) (32.7379, 15.7822) knots 0 0 0 1 2 2 2
  spline S131 degree 2 poles (32.7379, 15.7822) (32.7379, 15.7071) (32.7066, 15.524) knots 0 0 0 1 1 1
  line L231 (32.7066, 15.524) -> (32.5548, 14.6398)
  line L232 (32.5548, 14.6398) -> (32.2324, 14.6398)
  line L233 (32.2324, 14.6398) -> (32.3842, 15.5256)
  spline S132 degree 2 poles (32.3842, 15.5256) (32.4124, 15.6915) (32.4124, 15.7134) knots 0 0 0 1 1 1
  spline S133 degree 2 poles (32.4124, 15.7134) (32.4124, 15.776) (32.3482, 15.8433) (32.2934, 15.8433) knots 0 0 0 1 2 2 2
  spline S134 degree 2 poles (32.2934, 15.8433) (32.1745, 15.8433) (32.0806, 15.6993) knots 0 0 0 1 1 1
  spline S135 degree 2 poles (32.0806, 15.6993) (32.0055, 15.5851) (31.9554, 15.2987) knots 0 0 0 1 1 1
  line L234 (31.9554, 15.2987) -> (31.8427, 14.6398)
  line L235 (31.8427, 14.6398) -> (31.5204, 14.6398)
  line L236 (31.5204, 14.6398) -> (31.6706, 15.5162)
  spline S136 degree 2 poles (31.6706, 15.5162) (31.6956, 15.6664) (31.6956, 15.7103) knots 0 0 0 1 1 1
  spline S137 degree 2 poles (31.6956, 15.7103) (31.6956, 15.7729) (31.6283, 15.8433) (31.5751, 15.8433) knots 0 0 0 1 2 2 2
  spline S138 degree 2 poles (31.5751, 15.8433) (31.5047, 15.8433) (31.3529, 15.7103) (31.3091, 15.5835) knots 0 0 0 1 2 2 2
  spline S139 degree 2 poles (31.3091, 15.5835) (31.2825, 15.5084) (31.2465, 15.3049) knots 0 0 0 1 1 1
  line L237 (31.2465, 15.3049) -> (31.1307, 14.6398)
  line L238 (31.1307, 14.6398) -> (30.8083, 14.6398)
  line L239 (30.8083, 14.6398) -> (31.0571, 16.089)
  line L240 (33.8537, 14.6398) -> (33.5172, 14.6398)
  line L241 (33.5172, 14.6398) -> (33.8599, 16.6398)
  line L242 (33.8599, 16.6398) -> (34.5892, 16.6398)
  spline S140 degree 2 poles (34.5892, 16.6398) (34.7911, 16.6398) (34.9898, 16.5334) (35.1135, 16.2955) (35.1135, 16.114) knots 0 0 0 1 2 3 3 3
  spline S141 degree 2 poles (35.1135, 16.114) (35.1135, 15.848) (34.8537, 15.5272) (34.6095, 15.4896) knots 0 0 0 1 2 2 2
  spline S142 degree 2 poles (34.6095, 15.4896) (34.6768, 15.4145) (34.7426, 15.2768) knots 0 0 0 1 1 1
  spline S143 degree 2 poles (34.7426, 15.2768) (34.8505, 15.0452) (34.9804, 14.6398) knots 0 0 0 1 1 1
  line L243 (34.9804, 14.6398) -> (34.6189, 14.6398)
  spline S144 degree 2 poles (34.6189, 14.6398) (34.597, 14.7243) (34.4734, 15.0999) knots 0 0 0 1 1 1
  spline S145 degree 2 poles (34.4734, 15.0999) (34.4077, 15.2924) (34.3529, 15.3707) knots 0 0 0 1 1 1
  spline S146 degree 2 poles (34.3529, 15.3707) (34.3138, 15.427) (34.2308, 15.4677) (34.1338, 15.4677) knots 0 0 0 1 2 2 2
  line L244 (34.1338, 15.4677) -> (33.9961, 15.4677)
  line L245 (33.9961, 15.4677) -> (33.8537, 14.6398)
  line L246 (34.0462, 15.7682) -> (34.2261, 15.7682)
  spline S147 degree 2 poles (34.2261, 15.7682) (34.4797, 15.7682) (34.6581, 15.8323) (34.777, 16.0045) (34.777, 16.1078) knots 0 0 0 1 2 3 3 3
  spline S148 degree 2 poles (34.777, 16.1078) (34.777, 16.2204) (34.7019, 16.2721) knots 0 0 0 1 1 1
  spline S149 degree 2 poles (34.7019, 16.2721) (34.6581, 16.3049) (34.511, 16.3049) knots 0 0 0 1 1 1
  line L247 (34.511, 16.3049) -> (34.1385, 16.3049)
  line L248 (34.1385, 16.3049) -> (34.0462, 15.7682)
  line L249 (35.6127, 15.6774) -> (35.2997, 15.7103)
  spline S150 degree 2 poles (35.2997, 15.7103) (35.356, 15.9106) (35.633, 16.1218) (35.8459, 16.1218) knots 0 0 0 1 2 2 2
  spline S151 degree 2 poles (35.8459, 16.1218) (36.0634, 16.1218) (36.2966, 15.9074) (36.2966, 15.729) knots 0 0 0 1 2 2 2
  spline S152 degree 2 poles (36.2966, 15.729) (36.2966, 15.6664) (36.2746, 15.5256) (36.2042, 15.211) knots 0 0 0 1 2 2 2
  spline S153 degree 2 poles (36.2042, 15.211) (36.1448, 14.9513) (36.1448, 14.848) knots 0 0 0 1 1 1
  spline S154 degree 2 poles (36.1448, 14.848) (36.1448, 14.7525) (36.1776, 14.6398) knots 0 0 0 1 1 1
  line L250 (36.1776, 14.6398) -> (35.8568, 14.6398)
  spline S155 degree 2 poles (35.8568, 14.6398) (35.838, 14.7197) (35.8333, 14.8042) knots 0 0 0 1 1 1
  spline S156 degree 2 poles (35.8333, 14.8042) (35.7645, 14.7087) (35.5876, 14.607) (35.5, 14.607) knots 0 0 0 1 2 2 2
  spline S157 degree 2 poles (35.5, 14.607) (35.3607, 14.607) (35.1714, 14.8355) (35.1714, 15.0279) knots 0 0 0 1 2 2 2
  spline S158 degree 2 poles (35.1714, 15.0279) (35.1714, 15.247) (35.2825, 15.366) knots 0 0 0 1 1 1
  spline S159 degree 2 poles (35.2825, 15.366) (35.3936, 15.4849) (35.6534, 15.5084) knots 0 0 0 1 1 1
  spline S160 degree 2 poles (35.6534, 15.5084) (35.8834, 15.5319) (35.9601, 15.5647) knots 0 0 0 1 1 1
  spline S161 degree 2 poles (35.9601, 15.5647) (35.9867, 15.6477) (35.9867, 15.6962) knots 0 0 0 1 1 1
  spline S162 degree 2 poles (35.9867, 15.6962) (35.9867, 15.7619) (35.8959, 15.8433) (35.8192, 15.8433) knots 0 0 0 1 2 2 2
  spline S163 degree 2 poles (35.8192, 15.8433) (35.6502, 15.8433) (35.6127, 15.6774) knots 0 0 0 1 1 1
  spline S164 degree 2 poles (35.9085, 15.3143) (35.8787, 15.3049) (35.8318, 15.2971) knots 0 0 0 1 1 1
  spline S165 degree 2 poles (35.8318, 15.2971) (35.6127, 15.2643) (35.4734, 15.1531) (35.4734, 15.0608) knots 0 0 0 1 2 2 2
  spline S166 degree 2 poles (35.4734, 15.0608) (35.4734, 14.9888) (35.5532, 14.8996) (35.6142, 14.8996) knots 0 0 0 1 2 2 2
  spline S167 degree 2 poles (35.6142, 14.8996) (35.6768, 14.8996) (35.7942, 14.9747) (35.8631, 15.1093) (35.8959, 15.2627) knots 0 0 0 1 2 3 3 3
  line L251 (35.8959, 15.2627) -> (35.9085, 15.3143)
  line L252 (37.5063, 14.6398) -> (37.2011, 14.6398)
  line L253 (37.2011, 14.6398) -> (37.2293, 14.7963)
  spline S168 degree 2 poles (37.2293, 14.7963) (37.1432, 14.6915) (36.9773, 14.607) (36.8803, 14.607) knots 0 0 0 1 2 2 2
  spline S169 degree 2 poles (36.8803, 14.607) (36.7034, 14.607) (36.4781, 14.9106) (36.4781, 15.2142) knots 0 0 0 1 2 2 2
  spline S170 degree 2 poles (36.4781, 15.2142) (36.4781, 15.5725) (36.802, 16.1218) (37.0556, 16.1218) knots 0 0 0 1 2 2 2
  spline S171 degree 2 poles (37.0556, 16.1218) (37.2903, 16.1218) (37.4092, 15.8918) knots 0 0 0 1 1 1
  line L254 (37.4092, 15.8918) -> (37.5438, 16.6398)
  line L255 (37.5438, 16.6398) -> (37.8646, 16.6398)
  line L256 (37.8646, 16.6398) -> (37.5063, 14.6398)
  spline S172 degree 2 poles (36.7911, 15.2298) (36.7911, 15.0718) (36.9163, 14.8996) (37.0055, 14.8996) knots 0 0 0 1 2 2 2
  spline S173 degree 2 poles (37.0055, 14.8996) (37.079, 14.8996) (37.2183, 15.0186) (37.3216, 15.319) (37.3216, 15.4786) knots 0 0 0 1 2 3 3 3
  spline S174 degree 2 poles (37.3216, 15.4786) (37.3216, 15.6414) (37.187, 15.8339) (37.1009, 15.8339) knots 0 0 0 1 2 2 2
  spline S175 degree 2 poles (37.1009, 15.8339) (37.0336, 15.8339) (36.8944, 15.7103) (36.7911, 15.4004) (36.7911, 15.2298) knots 0 0 0 1 2 3 3 3
  line L257 (38.0822, 16.089) -> (38.403, 16.089)
  line L258 (38.403, 16.089) -> (38.1557, 14.6398)
  line L259 (38.1557, 14.6398) -> (37.8333, 14.6398)
  line L260 (37.8333, 14.6398) -> (38.0822, 16.089)
  line L261 (38.1761, 16.6398) -> (38.4984, 16.6398)
  line L262 (38.4984, 16.6398) -> (38.4374, 16.2862)
  line L263 (38.4374, 16.2862) -> (38.1166, 16.2862)
  line L264 (38.1166, 16.2862) -> (38.1761, 16.6398)
  spline S176 degree 2 poles (38.5188, 15.2423) (38.5188, 15.5976) (38.68, 15.848) knots 0 0 0 1 1 1
  spline S177 degree 2 poles (38.68, 15.848) (38.8584, 16.1218) (39.1964, 16.1218) knots 0 0 0 1 1 1
  spline S178 degree 2 poles (39.1964, 16.1218) (39.4499, 16.1218) (39.7519, 15.7776) (39.7519, 15.4708) knots 0 0 0 1 2 2 2
  spline S179 degree 2 poles (39.7519, 15.4708) (39.7519, 15.1109) (39.3764, 14.607) (39.0743, 14.607) knots 0 0 0 1 2 2 2
  spline S180 degree 2 poles (39.0743, 14.607) (38.8271, 14.607) (38.5188, 14.9481) (38.5188, 15.2423) knots 0 0 0 1 2 2 2
  spline S181 degree 2 poles (39.4343, 15.5225) (39.4343, 15.6649) (39.2997, 15.8292) (39.1948, 15.8292) knots 0 0 0 1 2 2 2
  spline S182 degree 2 poles (39.1948, 15.8292) (39.1072, 15.8292) (38.9538, 15.7087) (38.8396, 15.4114) (38.8396, 15.2517) knots 0 0 0 1 2 3 3 3
  spline S183 degree 2 poles (38.8396, 15.2517) (38.8396, 15.089) (38.9804, 14.909) (39.0837, 14.909) knots 0 0 0 1 2 2 2
  spline S184 degree 2 poles (39.0837, 14.909) (39.2152, 14.909) (39.3075, 15.0483) knots 0 0 0 1 1 1
  spline S185 degree 2 poles (39.3075, 15.0483) (39.4343, 15.2392) (39.4343, 15.5225) knots 0 0 0 1 1 1
  line L265 (41.1025, 14.6398) -> (40.8255, 14.6398)
  line L266 (40.8255, 14.6398) -> (40.5861, 16.089)
  line L267 (40.5861, 16.089) -> (40.9006, 16.089)
  line L268 (40.9006, 16.089) -> (40.9851, 15.4567)
  spline S186 degree 2 poles (40.9851, 15.4567) (41.018, 15.211) (41.0274, 15.1156) knots 0 0 0 1 1 1
  line L269 (41.0274, 15.1156) -> (41.0978, 15.2768)
  line L270 (41.0978, 15.2768) -> (41.1886, 15.4771)
  line L271 (41.1886, 15.4771) -> (41.4828, 16.089)
  line L272 (41.4828, 16.089) -> (41.8302, 16.089)
  line L273 (41.8302, 16.089) -> (41.1025, 14.6398)
  line L274 (42.2934, 16.0139) -> (41.9789, 16.0718)
  spline S187 degree 2 poles (41.9789, 16.0718) (42.0195, 16.3581) (42.3012, 16.6461) (42.5047, 16.6461) knots 0 0 0 1 2 2 2
  spline S188 degree 2 poles (42.5047, 16.6461) (42.7253, 16.6461) (42.9961, 16.355) (42.9961, 16.1093) knots 0 0 0 1 2 2 2
  spline S189 degree 2 poles (42.9961, 16.1093) (42.9961, 15.9184) (42.8959, 15.7369) knots 0 0 0 1 1 1
  spline S190 degree 2 poles (42.8959, 15.7369) (42.8224, 15.6038) (42.597, 15.3456) knots 0 0 0 1 1 1
  spline S191 degree 2 poles (42.597, 15.3456) (42.3904, 15.114) (42.3153, 14.9966) knots 0 0 0 1 1 1
  line L275 (42.3153, 14.9966) -> (42.885, 14.9966)
  line L276 (42.885, 14.9966) -> (42.8239, 14.6398)
  line L277 (42.8239, 14.6398) -> (41.8271, 14.6398)
  spline S192 degree 2 poles (41.8271, 14.6398) (41.8521, 14.8621) (41.9695, 15.0639) knots 0 0 0 1 1 1
  spline S193 degree 2 poles (41.9695, 15.0639) (42.0477, 15.2001) (42.3388, 15.5366) knots 0 0 0 1 1 1
  spline S194 degree 2 poles (42.3388, 15.5366) (42.5501, 15.7822) (42.608, 15.8777) knots 0 0 0 1 1 1
  spline S195 degree 2 poles (42.608, 15.8777) (42.6846, 16.006) (42.6846, 16.1124) knots 0 0 0 1 1 1
  spline S196 degree 2 poles (42.6846, 16.1124) (42.6846, 16.2173) (42.5845, 16.3394) (42.5125, 16.3394) knots 0 0 0 1 2 2 2
  spline S197 degree 2 poles (42.5125, 16.3394) (42.3451, 16.3394) (42.2934, 16.0139) knots 0 0 0 1 1 1
  line L278 (43.1291, 15.017) -> (43.4452, 15.017)
  line L279 (43.4452, 15.017) -> (43.3795, 14.6398)
  line L280 (43.3795, 14.6398) -> (43.0634, 14.6398)
  line L281 (43.0634, 14.6398) -> (43.1291, 15.017)
  line L282 (43.8677, 15.7885) -> (43.9272, 16.1375)
  spline S198 degree 2 poles (43.9272, 16.1375) (44.3451, 16.3581) (44.572, 16.6524) knots 0 0 0 1 1 1
  line L283 (44.572, 16.6524) -> (44.7676, 16.6524)
  line L284 (44.7676, 16.6524) -> (44.4202, 14.6398)
  line L285 (44.4202, 14.6398) -> (44.0978, 14.6398)
  line L286 (44.0978, 14.6398) -> (44.3372, 16.0264)
  spline S199 degree 2 poles (44.3372, 16.0264) (44.2386, 15.9481) (43.9742, 15.8167) (43.8677, 15.7885) knots 0 0 0 1 2 2 2
  line L287 (76.4295, 22.4899) -> (76.9915, 22.2716)
  spline S200 degree 2 poles (76.9915, 22.2716) (76.8606, 21.6851) (76.2495, 21.145) (75.8021, 21.145) knots 0 0 0 1 2 2 2
  spline S201 degree 2 poles (75.8021, 21.145) (75.2429, 21.145) (74.8937, 21.576) knots 0 0 0 1 1 1
  spline S202 degree 2 poles (74.8937, 21.576) (74.4927, 22.0752) (74.4927, 22.9236) knots 0 0 0 1 1 1
  spline S203 degree 2 poles (74.4927, 22.9236) (74.4927, 23.8184) (74.8964, 24.3258) knots 0 0 0 1 1 1
  spline S204 degree 2 poles (74.8964, 24.3258) (75.2483, 24.765) (75.8403, 24.765) knots 0 0 0 1 1 1
  spline S205 degree 2 poles (75.8403, 24.765) (76.3232, 24.765) (76.6478, 24.4349) knots 0 0 0 1 1 1
  spline S206 degree 2 poles (76.6478, 24.4349) (76.8797, 24.203) (76.9861, 23.742) knots 0 0 0 1 1 1
  line L288 (76.9861, 23.742) -> (76.4132, 23.5756)
  spline S207 degree 2 poles (76.4132, 23.5756) (76.3586, 23.8593) (76.0313, 24.1621) (75.8103, 24.1621) knots 0 0 0 1 2 2 2
  spline S208 degree 2 poles (75.8103, 24.1621) (75.4911, 24.1621) (75.0901, 23.6083) (75.0901, 22.97) knots 0 0 0 1 2 2 2
  spline S209 degree 2 poles (75.0901, 22.97) (75.0901, 22.3071) (75.4802, 21.7479) (75.7939, 21.7479) knots 0 0 0 1 2 2 2
  spline S210 degree 2 poles (75.7939, 21.7479) (76.0231, 21.7479) (76.3559, 22.1025) (76.4295, 22.4899) knots 0 0 0 1 2 2 2
  spline S211 degree 2 poles (77.3707, 22.9345) (77.3707, 23.5592) (77.7417, 24.3694) (78.3364, 24.765) (78.762, 24.765) knots 0 0 0 1 2 3 3 3
  spline S212 degree 2 poles (78.762, 24.765) (79.3785, 24.765) (80.1532, 23.8238) (80.1532, 22.9564) knots 0 0 0 1 2 2 2
  spline S213 degree 2 poles (80.1532, 22.9564) (80.1532, 22.0752) (79.744, 21.5815) knots 0 0 0 1 1 1
  spline S214 degree 2 poles (79.744, 21.5815) (79.3812, 21.145) (78.7647, 21.145) knots 0 0 0 1 1 1
  spline S215 degree 2 poles (78.7647, 21.145) (78.1427, 21.145) (77.7799, 21.576) knots 0 0 0 1 1 1
  spline S216 degree 2 poles (77.7799, 21.576) (77.3707, 22.0725) (77.3707, 22.9345) knots 0 0 0 1 1 1
  spline S217 degree 2 poles (77.9681, 22.9564) (77.9681, 22.3535) (78.4264, 21.7479) (78.7647, 21.7479) knots 0 0 0 1 2 2 2
  spline S218 degree 2 poles (78.7647, 21.7479) (79.1057, 21.7479) (79.5558, 22.348) (79.5558, 22.97) knots 0 0 0 1 2 2 2
  spline S219 degree 2 poles (79.5558, 22.97) (79.5558, 23.5783) (79.1193, 24.1621) (78.7647, 24.1621) knots 0 0 0 1 2 2 2
  spline S220 degree 2 poles (78.7647, 24.1621) (78.4128, 24.1621) (77.9681, 23.5729) (77.9681, 22.9564) knots 0 0 0 1 2 2 2
  line L289 (80.6006, 21.205) -> (80.6006, 24.705)
  line L290 (80.6006, 24.705) -> (81.4681, 24.705)
  line L291 (81.4681, 24.705) -> (81.9892, 22.3153)
  line L292 (81.9892, 22.3153) -> (82.502, 24.705)
  line L293 (82.502, 24.705) -> (83.375, 24.705)
  line L294 (83.375, 24.705) -> (83.375, 21.205)
  line L295 (83.375, 21.205) -> (82.8348, 21.205)
  line L296 (82.8348, 21.205) -> (82.8348, 23.963)
  line L297 (82.8348, 23.963) -> (82.2647, 21.205)
  line L298 (82.2647, 21.205) -> (81.7082, 21.205)
  line L299 (81.7082, 21.205) -> (81.1408, 23.963)
  line L300 (81.1408, 23.963) -> (81.1408, 21.205)
  line L301 (81.1408, 21.205) -> (80.6006, 21.205)
  line L302 (83.9397, 21.205) -> (83.9397, 24.705)
  line L303 (83.9397, 24.705) -> (84.8072, 24.705)
  line L304 (84.8072, 24.705) -> (85.3282, 22.3153)
  line L305 (85.3282, 22.3153) -> (85.8411, 24.705)
  line L306 (85.8411, 24.705) -> (86.714, 24.705)
  line L307 (86.714, 24.705) -> (86.714, 21.205)
  line L308 (86.714, 21.205) -> (86.1739, 21.205)
  line L309 (86.1739, 21.205) -> (86.1739, 23.963)
  line L310 (86.1739, 23.963) -> (85.6037, 21.205)
  line L311 (85.6037, 21.205) -> (85.0472, 21.205)
  line L312 (85.0472, 21.205) -> (84.4798, 23.963)
  line L313 (84.4798, 23.963) -> (84.4798, 21.205)
  line L314 (84.4798, 21.205) -> (83.9397, 21.205)
  point P0 (4.7786, 16.6743)
  point P1 (21.59, 1.27)
  point P2 (86.995, 24.765)
  point P3 (110.49, 1.27)
  point P4 (172.085, 24.765)
  constraints: 104 end point, 32 point on circle, 16 centre point, 8 midpoint, 5 other
extrude "Vysunutí2" add sketch "Náčrt2" along normal blind 0.0003 contours L12 A21 L25 A22 | L13 A8 L23 A11 L18 L20 L19 L22 L24 A20 | A9 L27 A23 L26 L16 L14 L21 L15 A10 L17 | L37 L40 L36 | L36 L40 L39 L38 L37 | L36 L41 L39 L40 | L40 L38 L39 | L43 L46 L42 | L42 L46 L45 L44 L43 | L42 L47 L45 L46 | L46 L44 L45 | L49 L52 L48 | L48 L52 L51 L50 L49 | L48 L53 L51 L52 | L52 L50 L51 | L55 L58 L54 | L54 L58 L57 L56 L55 | L54 L59 L57 L58 | L58 L56 L57 | L60 L61 L62 L63 L64 L65 L66 L67 L68 L69 | L70 L71 L72 L73 L74 L75 L76 L77 | L81 L82 L83 L84 L85 L86 L87 | L88 L89 L90 L91 | L92 S0 S1 L93 L94 | L98 L99 L100 L101 L102 L103 L104 L105 L106 L107 L108 L109 | L110 L111 L112 L113 L114 L115 L116 L117 L118 L119 | L120 L121 L122 L123 L124 L125 L126 L127 | L128 L129 L130 L131 L132 L133 L134 L135 | L136 L137 L138 L139 L140 L141 L142 L143 L144 L145 L146 L147 | L148 S5 S6 S7 S8 S9 S10 L149 S11 S12 S13 S14 S15 S16 S17 | L150 L151 L152 L153 L154 L155 L156 L157 | L158 L159 L160 L161 L162 L163 L164 | L165 L166 S18 S19 L167 S20 S21 S22 S23 S24 | L170 L171 S27 S28 L172 S29 S30 S31 L173 L174 L175 | L176 L177 L178 S32 S33 S34 S35 L179 L180 | L181 S40 S41 S42 S43 S44 L182 S45 S46 S47 S48 S49 S50 S51 S52 S53 | L184 S58 S59 S60 S61 L185 S62 S63 S64 S65 | S66 S67 S68 S69 S70 | L186 L187 S76 S77 L188 S78 S79 S80 L189 L190 L191 | L192 L193 S81 S82 S83 S84 S85 L194 L195 L196 | L197 L198 L199 L200 | L201 L202 L203 L204 L205 L206 L207 L208 L209 L210 | L211 S90 S91 S92 S93 S94 L212 S95 S96 S97 S98 S99 S100 S101 S102 S103 | L214 L215 L216 L217 S108 L218 L219 L220 L221 L222 | L223 L224 L225 L226 | L227 S109 S110 S111 S112 L228 S113 S114 S115 S116 | S117 S118 S119 S120 S121 | L229 L230 S127 S128 S129 S130 S131 L231 L232 L233 S132 S133 S134 S135 L234 L235 L236 S136 S137 S138 S139 L237 L238 L239 | L240 L241 L242 S140 S141 S142 S143 L243 S144 S145 S146 L244 L245 | L249 S150 S151 S152 S153 S154 L250 S155 S156 S157 S158 S159 S160 S161 S162 S163 | L252 L253 S168 S169 S170 S171 L254 L255 L256 | L257 L258 L259 L260 | L261 L262 L263 L264 | S176 S177 S178 S179 S180 | L265 L266 L267 L268 S186 L269 L270 L271 L272 L273 | L274 S187 S188 S189 S190 S191 L275 L276 L277 S192 S193 S194 S195 S196 S197 | L278 L279 L280 L281 | L282 S198 L283 L284 L285 L286 S199 | L287 S200 S201 S202 S203 S204 S205 S206 L288 S207 S208 S209 S210 | S211 S212 S213 S214 S215 S216 | L289 L290 L291 L292 L293 L294 L295 L296 L297 L298 L299 L300 L301 | L302 L303 L304 L305 L306 L307 L308 L309 L310 L311 L312 L313 L314
